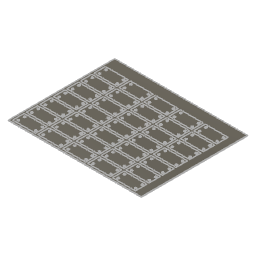
JSM-01 v4 (Autodesk Fusion 360 design; units mm, degrees)
Autodesk Fusion 360 part; units mm, degrees
sketch "Sketch1" plane through (0, 0, 0) normal (0, 0, 1) x (1, 0, 0)
  line L0 (0, 0) -> (500, 0)
  line L1 (500, 0) -> (500, 400)
  line L2 (500, 400) -> (0, 400)
  line L3 (0, 400) -> (0, 0)
  line L4 (8, 8) -> (94, 8)
  line L5 (94, 8) -> (94, 51)
  line L6 (94, 51) -> (8, 51)
  line L7 (8, 51) -> (8, 8)
  line L8 (8, 59) -> (94, 59)
  line L9 (8, 102) -> (8, 59)
  line L10 (94, 102) -> (8, 102)
  line L11 (94, 59) -> (94, 102)
  line L12 (94, 153) -> (8, 153)
  line L13 (8, 153) -> (8, 110)
  line L14 (8, 110) -> (94, 110)
  line L15 (94, 110) -> (94, 153)
  line L16 (94, 204) -> (8, 204)
  line L17 (8, 204) -> (8, 161)
  line L18 (8, 161) -> (94, 161)
  line L19 (94, 161) -> (94, 204)
  line L20 (94, 255) -> (8, 255)
  line L21 (8, 255) -> (8, 212)
  line L22 (8, 212) -> (94, 212)
  line L23 (94, 212) -> (94, 255)
  line L24 (94, 306) -> (8, 306)
  line L25 (8, 306) -> (8, 263)
  line L26 (8, 263) -> (94, 263)
  line L27 (94, 263) -> (94, 306)
  line L28 (94, 357) -> (8, 357)
  line L29 (8, 357) -> (8, 314)
  line L30 (8, 314) -> (94, 314)
  line L31 (94, 314) -> (94, 357)
  line L32 (102, 212) -> (188, 212)
  line L33 (102, 357) -> (102, 314)
  line L34 (102, 110) -> (188, 110)
  line L35 (188, 314) -> (188, 357)
  line L36 (188, 59) -> (188, 102)
  line L37 (188, 110) -> (188, 153)
  line L38 (102, 306) -> (102, 263)
  line L39 (188, 255) -> (102, 255)
  line L40 (188, 263) -> (188, 306)
  line L41 (188, 8) -> (188, 51)
  line L42 (188, 357) -> (102, 357)
  line L43 (102, 8) -> (188, 8)
  line L44 (102, 161) -> (188, 161)
  line L45 (188, 212) -> (188, 255)
  line L46 (102, 204) -> (102, 161)
  line L47 (102, 255) -> (102, 212)
  line L48 (102, 263) -> (188, 263)
  line L49 (188, 306) -> (102, 306)
  line L50 (188, 204) -> (102, 204)
  line L51 (102, 51) -> (102, 8)
  line L52 (102, 153) -> (102, 110)
  line L53 (188, 153) -> (102, 153)
  line L54 (188, 102) -> (102, 102)
  line L55 (102, 59) -> (188, 59)
  line L56 (102, 102) -> (102, 59)
  line L57 (102, 314) -> (188, 314)
  line L58 (188, 161) -> (188, 204)
  line L59 (188, 51) -> (102, 51)
  line L60 (196, 212) -> (282, 212)
  line L61 (196, 357) -> (196, 314)
  line L62 (196, 110) -> (282, 110)
  line L63 (282, 314) -> (282, 357)
  line L64 (282, 59) -> (282, 102)
  line L65 (282, 110) -> (282, 153)
  line L66 (196, 306) -> (196, 263)
  line L67 (282, 255) -> (196, 255)
  line L68 (282, 263) -> (282, 306)
  line L69 (282, 8) -> (282, 51)
  line L70 (282, 357) -> (196, 357)
  line L71 (196, 8) -> (282, 8)
  line L72 (196, 161) -> (282, 161)
  line L73 (282, 212) -> (282, 255)
  line L74 (196, 204) -> (196, 161)
  line L75 (196, 255) -> (196, 212)
  line L76 (196, 263) -> (282, 263)
  line L77 (282, 306) -> (196, 306)
  line L78 (282, 204) -> (196, 204)
  line L79 (196, 51) -> (196, 8)
  line L80 (196, 153) -> (196, 110)
  line L81 (282, 153) -> (196, 153)
  line L82 (282, 102) -> (196, 102)
  line L83 (196, 59) -> (282, 59)
  line L84 (196, 102) -> (196, 59)
  line L85 (196, 314) -> (282, 314)
  line L86 (282, 161) -> (282, 204)
  line L87 (282, 51) -> (196, 51)
  line L88 (290, 212) -> (376, 212)
  line L89 (290, 357) -> (290, 314)
  line L90 (290, 110) -> (376, 110)
  line L91 (376, 314) -> (376, 357)
  line L92 (376, 59) -> (376, 102)
  line L93 (376, 110) -> (376, 153)
  line L94 (290, 306) -> (290, 263)
  line L95 (376, 255) -> (290, 255)
  line L96 (376, 263) -> (376, 306)
  line L97 (376, 8) -> (376, 51)
  line L98 (376, 357) -> (290, 357)
  line L99 (290, 8) -> (376, 8)
  line L100 (290, 161) -> (376, 161)
  line L101 (376, 212) -> (376, 255)
  line L102 (290, 204) -> (290, 161)
  line L103 (290, 255) -> (290, 212)
  line L104 (290, 263) -> (376, 263)
  line L105 (376, 306) -> (290, 306)
  line L106 (376, 204) -> (290, 204)
  line L107 (290, 51) -> (290, 8)
  line L108 (290, 153) -> (290, 110)
  line L109 (376, 153) -> (290, 153)
  line L110 (376, 102) -> (290, 102)
  line L111 (290, 59) -> (376, 59)
  line L112 (290, 102) -> (290, 59)
  line L113 (290, 314) -> (376, 314)
  line L114 (376, 161) -> (376, 204)
  line L115 (376, 51) -> (290, 51)
  line L116 (384, 212) -> (470, 212)
  line L117 (384, 357) -> (384, 314)
  line L118 (384, 110) -> (470, 110)
  line L119 (470, 314) -> (470, 357)
  line L120 (470, 59) -> (470, 102)
  line L121 (470, 110) -> (470, 153)
  line L122 (384, 306) -> (384, 263)
  line L123 (470, 255) -> (384, 255)
  line L124 (470, 263) -> (470, 306)
  line L125 (470, 8) -> (470, 51)
  line L126 (470, 357) -> (384, 357)
  line L127 (384, 8) -> (470, 8)
  line L128 (384, 161) -> (470, 161)
  line L129 (470, 212) -> (470, 255)
  line L130 (384, 204) -> (384, 161)
  line L131 (384, 255) -> (384, 212)
  line L132 (384, 263) -> (470, 263)
  line L133 (470, 306) -> (384, 306)
  line L134 (470, 204) -> (384, 204)
  line L135 (384, 51) -> (384, 8)
  line L136 (384, 153) -> (384, 110)
  line L137 (470, 153) -> (384, 153)
  line L138 (470, 102) -> (384, 102)
  line L139 (384, 59) -> (470, 59)
  line L140 (384, 102) -> (384, 59)
  line L141 (384, 314) -> (470, 314)
  line L142 (470, 161) -> (470, 204)
  line L143 (470, 51) -> (384, 51)
  constraint horizontal L0
  constraint vertical L1
  constraint horizontal L2
  constraint vertical L3
  constraint coincident L0.start L3.end
  constraint horizontal L4
  constraint vertical L5
  constraint horizontal L6
  constraint vertical L7
  constraint horizontal L8
  constraint vertical L11
  constraint horizontal L10
  constraint vertical L9
  constraint horizontal L14
  constraint vertical L15
  constraint horizontal L12
  constraint vertical L13
  constraint horizontal L18
  constraint vertical L19
  constraint horizontal L16
  constraint vertical L17
  constraint horizontal L22
  constraint vertical L23
  constraint horizontal L20
  constraint vertical L21
  constraint horizontal L26
  constraint vertical L27
  constraint horizontal L24
  constraint vertical L25
  constraint horizontal L30
  constraint vertical L31
  constraint horizontal L28
  constraint vertical L29
  constraint horizontal L43
  constraint vertical L41
  constraint horizontal L59
  constraint vertical L51
  constraint horizontal L55
  constraint vertical L36
  constraint horizontal L54
  constraint vertical L56
  constraint horizontal L34
  constraint vertical L37
  constraint horizontal L53
  constraint vertical L52
  constraint horizontal L44
  constraint vertical L58
  constraint horizontal L50
  constraint vertical L46
  constraint horizontal L32
  constraint vertical L45
  constraint horizontal L39
  constraint vertical L47
  constraint horizontal L48
  constraint vertical L40
  constraint horizontal L49
  constraint vertical L38
  constraint horizontal L57
  constraint vertical L35
  constraint horizontal L42
  constraint vertical L33
  constraint horizontal L71
  constraint vertical L69
  constraint horizontal L87
  constraint vertical L79
  constraint horizontal L83
  constraint vertical L64
  constraint horizontal L82
  constraint vertical L84
  constraint horizontal L62
  constraint vertical L65
  constraint horizontal L81
  constraint vertical L80
  constraint horizontal L72
  constraint vertical L86
  constraint horizontal L78
  constraint vertical L74
  constraint horizontal L60
  constraint vertical L73
  constraint horizontal L67
  constraint vertical L75
  constraint horizontal L76
  constraint vertical L68
  constraint horizontal L77
  constraint vertical L66
  constraint horizontal L85
  constraint vertical L63
  constraint horizontal L70
  constraint vertical L61
  constraint horizontal L99
  constraint vertical L97
  constraint horizontal L115
  constraint vertical L107
  constraint horizontal L111
  constraint vertical L92
  constraint horizontal L110
  constraint vertical L112
  constraint horizontal L90
  constraint vertical L93
  constraint horizontal L109
  constraint vertical L108
  constraint horizontal L100
  constraint vertical L114
  constraint horizontal L106
  constraint vertical L102
  constraint horizontal L88
  constraint vertical L101
  constraint horizontal L95
  constraint vertical L103
  constraint horizontal L104
  constraint vertical L96
  constraint horizontal L105
  constraint vertical L94
  constraint horizontal L113
  constraint vertical L91
  constraint horizontal L98
  constraint vertical L89
  constraint horizontal L127
  constraint vertical L125
  constraint horizontal L143
  constraint vertical L135
  constraint horizontal L139
  constraint vertical L120
  constraint horizontal L138
  constraint vertical L140
  constraint horizontal L118
  constraint vertical L121
  constraint horizontal L137
  constraint vertical L136
  constraint horizontal L128
  constraint vertical L142
  constraint horizontal L134
  constraint vertical L130
  constraint horizontal L116
  constraint vertical L129
  constraint horizontal L123
  constraint vertical L131
  constraint horizontal L132
  constraint vertical L124
  constraint horizontal L133
  constraint vertical L122
  constraint horizontal L141
  constraint vertical L119
  constraint horizontal L126
  constraint vertical L117
extrude "Extrude8" add sketch "Sketch1" along normal blind 2 makes body 1
sketch "Sketch2" plane through (0, 0, 0) normal (0, 0, 1) x (1, 0, 0)
  line L0 (0, 0) -> (86, 0)
  line L1 (86, 0) -> (86, 43)
  line L2 (86, 43) -> (0, 43)
  line L3 (0, 43) -> (0, 0)
  circle A0 centre (11.5, 33.5) radius 3.75
  circle A1 centre (78, 33.5) radius 3.75
  circle A2 centre (11.5, 9.5) radius 3.75
  circle A3 centre (78, 9.5) radius 3.75
  constraint horizontal L0
  constraint vertical L1
  constraint horizontal L2
  constraint vertical L3
  constraint coincident L0.start L3.end
extrude "Extrude9" add sketch "Sketch2" along normal blind 2 separate body makes body 2
move_body "Move21" bodies 2 to x (1, 0, 0) y (0, 1, 0) z (0, 0, 1) at (8, 8, 0)
copy_body "CopyPasteBodies19" bodies 2 makes body 3
move_body "Move22" bodies 3 to x (1, 0, 0) y (0, 1, 0) z (0, 0, 1) at (0, 51, 0)
copy_body "CopyPasteBodies20" bodies 2 makes body 4
move_body "Move23" bodies 4 to x (1, 0, 0) y (0, 1, 0) z (0, 0, 1) at (0, 102, 0)
copy_body "CopyPasteBodies22" bodies 2 makes body 5
move_body "Move24" bodies 5 to x (1, 0, 0) y (0, 1, 0) z (0, 0, 1) at (0, 153, 0)
copy_body "CopyPasteBodies23" bodies 2 makes body 6
move_body "Move25" bodies 6 to x (1, 0, 0) y (0, 1, 0) z (0, 0, 1) at (0, 204, 0)
copy_body "CopyPasteBodies24" bodies 2 makes body 7
move_body "Move26" bodies 7 to x (1, 0, 0) y (0, 1, 0) z (0, 0, 1) at (0, 255, 0)
copy_body "CopyPasteBodies25" bodies 2 makes body 8
move_body "Move27" bodies 8 to x (1, 0, 0) y (0, 1, 0) z (0, 0, 1) at (0, 306, 0)
copy_body "CopyPasteBodies26" bodies 5 3 6 2 4 8 7 makes body 9 makes body 10 makes body 11 makes body 12 makes body 13 makes body 14 makes body 15
move_body "Move28" bodies 9 10 11 12 13 14 15 to x (1, 0, 0) y (0, 1, 0) z (0, 0, 1) at (94, 0, 0)
copy_body "CopyPasteBodies27" bodies 5 3 6 2 4 8 7 makes body 16 makes body 17 makes body 18 makes body 19 makes body 20 makes body 21 makes body 22
move_body "Move29" bodies 16 17 18 19 20 21 22 to x (1, 0, 0) y (0, 1, 0) z (0, 0, 1) at (188, 0, 0)
copy_body "CopyPasteBodies28" bodies 5 3 6 2 4 8 7 makes body 23 makes body 24 makes body 25 makes body 26 makes body 27 makes body 28 makes body 29
move_body "Move30" bodies 23 24 25 26 27 28 29 to x (1, 0, 0) y (0, 1, 0) z (0, 0, 1) at (282, 0, 0)
copy_body "CopyPasteBodies29" bodies 5 3 6 2 4 8 7 makes body 30 makes body 31 makes body 32 makes body 33 makes body 34 makes body 35 makes body 36
move_body "Move31" bodies 30 31 32 33 34 35 36 to x (1, 0, 0) y (0, 1, 0) z (0, 0, 1) at (376, 0, 0)
named bodies: "Body1", "Body2", "Body3", "Body2 (1)", "Body4", "Body2 (3)", "Body5", "Body2 (4)", "Body6", "Body2 (5)", "Body7", "Body2 (2)", "Body8", "Body2 (6)", "Body5 (1)", "Body3 (1)", "Body6 (1)", "Body4 (1)", "Body8 (1)", "Body7 (1)", "Body2 (7)", "Body5 (2)", "Body3 (2)", "Body6 (2)", "Body4 (2)", "Body8 (2)", "Body7 (2)", "Body2 (8)", "Body5 (3)", "Body3 (3)", "Body6 (3)", "Body4 (3)", "Body8 (3)", "Body7 (3)", "Body2 (9)", "Body5 (4)", "Body3 (4)", "Body6 (4)", "Body4 (4)", "Body8 (4)", "Body7 (4)"
